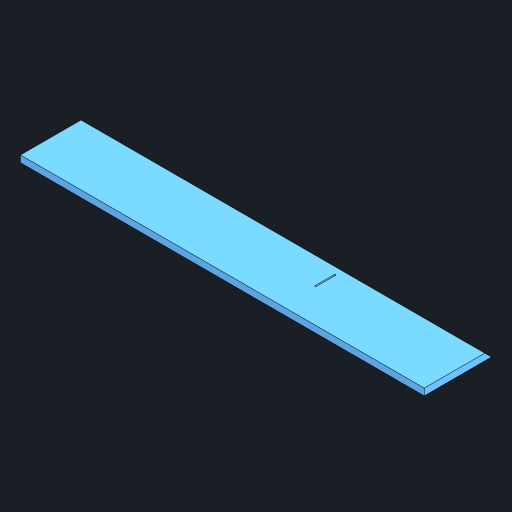
# Autodesk Inventor part: HoriMove
Saved by Autodesk Inventor 2023 (Build 270158000, 158)
## iProperties
Created: 2022-06-07
Part Number: HoriMove
Material: スタイロフォームIB
Document SubType Name: Modeling
Designer: neko2
Density: 0.027 g/cm^3
Appearance: スタイロフォームIB
Mass: 1.08675 g
Surface Area: 183.649 cm^2
Volume: 40.25 cm^3
Author: neko2
Autodesk Inventor part; units mm, degrees
ref_plane "YZ Plane" through (0, 0, 0) normal (1, 0, 0) x (0, 1, 0)
ref_plane "XZ Plane" through (0, 0, 0) normal (0, 1, 0) x (-1, 0, 0)
ref_plane "XY Plane" through (0, 0, 0) normal (0, 0, 1) x (1, 0, 0)
sketch "スケッチ1" plane through (0, 0, 0) normal (0, 1, 0) x (-1, 0, 0)
  line L0 (150, -25) -> (-150, -25)
  line L1 (-150, -25) -> (-150, 25)
  line L2 (-150, 25) -> (150, 25)
  line L3 (150, 25) -> (150, -25)
  line L4 (150, -25) -> (-150, 25) construction
  line L5 (-150, -25) -> (150, 25) construction
  line L6 (150, -25) -> (70, -25)
  line L7 (70, -25) -> (70, -60)
  line L8 (70, -60) -> (150, -60)
  line L9 (150, -60) -> (150, -25)
  line L10 (0, 25) -> (0, -116.583)
  line L11 (-70, -25) -> (-70, -60)
  line L12 (-70, -60) -> (-150, -60)
  line L13 (-150, -60) -> (-150, -25)
  point P0 (0, 0)
  dimension "d0" = 300
  dimension "d1" = 50
  dimension "d7" = 80
  dimension "d8" = 35
  constraints: 28 end point, 4 parallel, 3 midpoint, 3 symmetric about line, 2 horizontal, 2 perpendicular, 1 vertical
  measures "d0" distance of L1.end L2.end
  measures "d1" distance of L0.end L1.end
  measures "d7" distance of L8.end L7.end
  measures "d8" distance of L7.end L6.end
extrude "押し出し1" add sketch "スケッチ1" along normal blind 5 contours L0 L10 L2 L3 | L0 L1 L2 L10
chamfer "面取り1" distance 5 angle 45 1 edges at (0, 5, -25)
sketch "スケッチ4" plane through (0, 5, 0) normal (0, 1, 0) x (1, 0, 0)
  line L0 (48, 20) -> (40, 20)
  line L1 (40, 20) -> (40, -5)
  line L2 (40, -5) -> (48, -5)
  line L3 (48, -5) -> (48, 20)
  line L4 (43.5, 0) -> (44.5, 0)
  line L5 (44.5, 0) -> (44.5, 15)
  line L6 (44.5, 15) -> (43.5, 15)
  line L7 (43.5, 15) -> (43.5, 0)
  line L8 (-150, 20) -> (150, 20) projected
  point P0 (0, 0)
  point P1 (44, 0)
  point P2 (44, -5)
  point P3 (43.5, 7.5)
  point P4 (40, 7.5)
  dimension "d12" = 8
  dimension "d13" = 25
  dimension "d14" = 1
  dimension "d15" = 15
  dimension "d22" = 40
  constraints: 16 end point, 4 midpoint, 4 parallel, 2 horizontal, 2 perpendicular, 1 horizontal alignment, 1 point on line, 1 vertical alignment
  measures "d12" distance of L2.end L1.end
  measures "d13" distance of L1.end L0.end
  measures "d14" distance of L5.end L6.end
  measures "d15" distance of L6.end L4.start
  measures "d22" distance from line of point (0, 0) L1
extrude "押し出し4" cut sketch "スケッチ4" against normal through all contours L7 L6 L5 L4
